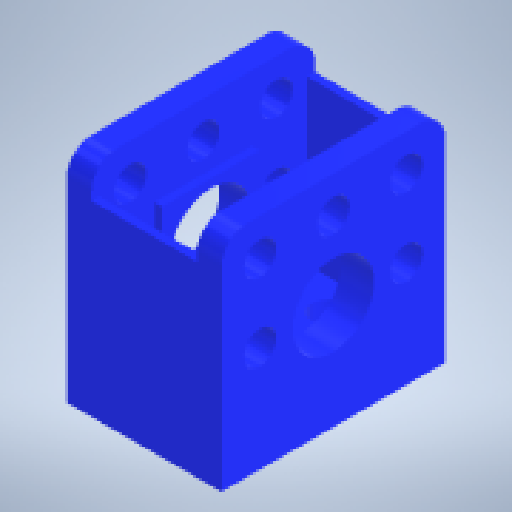
# Autodesk Inventor part: SoporteEncoder
Saved by Autodesk Inventor 2023.1 (Build 271208000, 208)
## iProperties
Created: 2023-05-02
Part Number: SoporteEncoder
Material: Plastic, Opaque Black
Document SubType Name: Modeling
Designer: felip
Density: 0.952 g/cm^3
Appearance: Blue - Wall Paint - Glossy
Author: felip
Autodesk Inventor part; units mm, degrees
ref_plane "YZ Plane" through (0, 0, 0) normal (1, 0, 0) x (0, 1, 0)
ref_plane "XZ Plane" through (0, 0, 0) normal (0, 1, 0) x (-1, 0, 0)
ref_plane "XY Plane" through (0, 0, 0) normal (0, 0, 1) x (1, 0, 0)
sketch "Sketch1" plane through (0, 0, 0) normal (0, 1, 0) x (-1, 0, 0)
  line L0 (9.5, 13.75) -> (-9.5, 13.75)
  line L1 (-9.5, 13.75) -> (-9.5, -13.75)
  line L2 (-9.5, -13.75) -> (9.5, -13.75)
  line L3 (9.5, -13.75) -> (9.5, 13.75)
  point P0 (0, 0)
  dimension "d0" = 19
  dimension "d1" = 27.5
  dimension "d2" = 13.75
  dimension "d3" = 9.5
  constraints: 8 end point, 2 parallel, 1 horizontal, 1 perpendicular
  measures "d0" distance of L0.start L0.end
  measures "d1" distance of L2.end L0.start
  measures "d2" distance from line of L0 point (0, 0)
  measures "d3" distance from line of point (0, 0) L3
extrude "Extrusion1" add sketch "Sketch1" along normal blind 27
sketch "Sketch2" plane through (0, 27, 0) normal (0, 1, 0) x (1, 0, 0)
  line L0 (9.5, 13.75) -> (-9.5, 13.75) projected
  line L1 (9.5, -13.75) -> (9.5, 13.75) projected
  line L2 (-9.5, -13.75) -> (9.5, -13.75) projected
  line L3 (-9.5, 13.75) -> (-9.5, -13.75) projected
  line L4 (-6.5, -12.75) -> (6.5, -12.75)
  line L5 (6.5, -12.75) -> (6.5, 12.75)
  line L6 (6.5, 12.75) -> (-6.5, 12.75)
  line L7 (-6.5, 12.75) -> (-6.5, -12.75)
  point P0 (0, 0)
  dimension "d6" = 3
  dimension "d7" = 3
  dimension "d8" = 1
  dimension "d9" = 1
  constraints: 8 end point, 2 parallel, 1 horizontal, 1 perpendicular
  measures "d6" distance between parallel lines of L1 L5
  measures "d7" distance between parallel lines of L3 L7
  measures "d8" distance between parallel lines of L0 L6
  measures "d9" distance between parallel lines of L2 L4
extrude "Extrusion2" cut sketch "Sketch2" against normal blind 24 contours L7 L6 L5 L4
sketch "Sketch3" plane through (-9.5, 0, 13.75) normal (0, 0, 1) x (1, 0, 0)
  line L0 (0, 27) -> (19, 27) projected
  line L1 (3, 27) -> (3, 3) projected
  line L2 (16, 27) -> (16, 3) projected
  line L3 (3, 27) -> (3, 3) projected
  line L4 (16, 27) -> (16, 3) projected
  line L5 (3, 27) -> (16, 27)
  line L6 (16, 27) -> (16, 23)
  line L7 (16, 23) -> (3, 23)
  line L8 (3, 23) -> (3, 27)
  point P0 (9.5, 0)
  point P1 (3, 23)
  dimension "d12" = 4
  constraints: 8 end point, 2 parallel, 1 horizontal, 1 perpendicular, 1 point on line
  measures "d12" distance between parallel lines of L7 L0
extrude "Extrusion3" cut sketch "Sketch3" against normal blind 30
fillet "Fillet1" radius 3 4 edges at (-8, 27, 13.75) (-8, 27, -13.75) (8, 27, -13.75) (8, 27, 13.75)
sketch "Sketch4" plane through (0, 0, 0) normal (0, -1, 0) x (1, 0, 0)
  circle A0 centre (0, 0) radius 2
  circle A1 centre (0, -9) radius 2
  circle A2 centre (0, 9) radius 2
  dimension "d16" = 4
  dimension "d17" = 4
  dimension "d18" = 4
  dimension "d19" = 9
  dimension "d20" = 9
  constraints: 3 centre point, 1 coincident
  measures "d16" diameter of A0
  measures "d17" diameter of A1
  measures "d18" diameter of A2
  measures "d19" distance of A1.centre point (0, 0)
  measures "d20" distance of point (0, 0) A2.centre
extrude "Extrusion4" cut sketch "Sketch4" against normal blind 5
sketch "Sketch5" plane through (9.5, 0, 13.75) normal (1, 0, 0) x (0, 0, -1)
  line L0 (3, 27) -> (24.5, 27) projected
  line L1 (27.5, 0) -> (27.5, 24) projected
  line L2 (0, 0) -> (0, 24) projected
  circle A0 centre (13.75, 13) radius 2
  circle A1 centre (22.75, 13) radius 2
  circle A2 centre (4.75, 13) radius 2
  line L3 (1.7351, 17.75) -> (24.75, 17.75) construction
  circle A3 centre (13.75, 22.5) radius 2
  circle A4 centre (22.75, 22.5) radius 2
  circle A5 centre (4.75, 22.5) radius 2
  point P0 (13.75, 0)
  dimension "d23" = 14
  dimension "d24" = 27.5
  dimension "d25" = 13.75
  dimension "d26" = 4
  dimension "d27" = 0
  dimension "d28" = 0
  dimension "d29" = 4
  dimension "d30" = 4
  dimension "d31" = 9
  dimension "d32" = 9
  dimension "d35" = 4.75
  constraints: 6 centre point, 3 symmetric about line, 2 end point, 1 horizontal, 3 other
  measures "d23" distance from line of A0.centre L0
  measures "d24" distance between parallel lines of L1 L2
  measures "d25" distance from line of L2 A0.centre
  measures "d26" diameter of A0
  measures "d27" vertical distance of A0.centre A2.centre
  measures "d28" vertical distance of A0.centre A1.centre
  measures "d29" diameter of A1
  measures "d30" diameter of A2
  measures "d31" distance of A0.centre A2.centre
  measures "d32" distance of A0.centre A1.centre
  measures "d35" distance from line of A0.centre L3
hole "Hole1" at (9.5, 22.5, 9) at (9.5, 22.5, 0) at (9.5, 22.5, -9) at (9.5, 13, 0) at (9.5, 13, -9) at (9.5, 13, 9) direction (-1, 0, 0) diameter 4 end through all
sketch "Sketch6" plane through (-6.5, 3, 12.75) normal (1, 0, 0) x (0, 0, -1)
  circle A0 centre (12.75, 10) radius 2 projected
  line L0 (6.75, 16) -> (18.75, 16)
  line L1 (18.75, 16) -> (18.75, 4)
  line L2 (18.75, 4) -> (6.75, 4)
  line L3 (6.75, 4) -> (6.75, 16)
  point P0 (12.75, -3)
  dimension "d43" = 12
  dimension "d44" = 12
  dimension "d45" = 6
  dimension "d46" = 6
  constraints: 8 end point, 2 parallel, 1 horizontal, 1 perpendicular
  measures "d43" distance of L0.start L0.end
  measures "d44" distance of L0.end L1.end
  measures "d45" distance from line of L1 A0.centre
  measures "d46" distance from line of L0 A0.centre
extrude "Extrusion5" add sketch "Sketch6" along normal blind 1
sketch "Sketch7" plane through (6.5, 3, -12.75) normal (-1, 0, 0) x (0, 0, 1)
  line L0 (6.75, 16) -> (18.75, 16) projected
  line L1 (6.75, 4) -> (6.75, 16) projected
  line L2 (18.75, 16) -> (18.75, 4) projected
  line L3 (18.75, 4) -> (6.75, 4) projected
  circle A0 centre (12.75, 10) radius 2 projected
  line L4 (18.75, 16) -> (6.75, 16)
  line L5 (6.75, 16) -> (6.75, 4)
  line L6 (6.75, 4) -> (18.75, 4)
  line L7 (18.75, 4) -> (18.75, 16)
  point P0 (12.75, -3)
  constraints: 8 end point, 2 parallel, 1 horizontal, 1 perpendicular
extrude "Extrusion6" add sketch "Sketch7" along normal blind 1
sketch "Sketch8" plane through (-9.5, 0, -13.75) normal (-1, 0, 0) x (0, 0, 1)
  circle A0 centre (13.75, 13) radius 2 projected
  circle A1 centre (13.75, 13) radius 5
  point P0 (13.75, 0)
  dimension "d51" = 10
  constraints: 1 centre point, 1 coincident
  measures "d51" diameter of A1
extrude "Extrusion7" cut sketch "Sketch8" against normal through all
equation "\"d2\" = 0.5 * d1"
equation "\"d3\" = 0.5 * d0"
equation "\"d16\" = d17"
equation "\"d18\" = d17"
equation "\"d20\" = d19"
equation "\"d25\" = 0.5 * d24"
equation "\"d29\" = d26"
equation "\"d30\" = d26"
body "Solid1"
